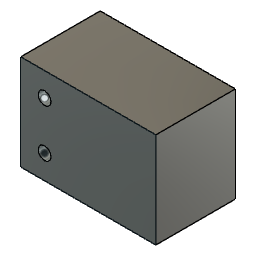
X-AxisLimitSwitchBlock v2 (Autodesk Fusion 360 design; units mm, degrees)
Autodesk Fusion 360 part; units mm, degrees
sketch "Sketch1" plane through (0, 0, 0) normal (0, 1, 0) x (1, 0, 0)
  line L0 (0, 0) -> (17, 0)
  line L1 (17, 0) -> (17, -10)
  line L2 (17, -10) -> (0, -10)
  line L3 (0, -10) -> (0, 0)
  dimension "d1" = 17
  dimension "d2" = 10
  constraint horizontal L0
  constraint vertical L1
  constraint horizontal L2
  constraint vertical L3
  constraint coincident L0.start L3.end
  measures "d1" distance of L0.start L0.end
  measures "d2" distance of L0.start L2.end
extrude "Extrude1" add sketch "Sketch1" along normal blind 12
sketch "Sketch2" plane through (0, 0, 10) normal (0, 0, 1) x (1, 0, 0)
  line L0 (0, 0) -> (17, 0)
  line L1 (17, 0) -> (17, 12)
  line L2 (17, 12) -> (0, 12)
  line L3 (0, 12) -> (0, 0)
  point P0 (3, 3)
  point P1 (3, 9)
  dimension "d5" = 3
  dimension "d6" = 3
  dimension "d7" = 6
  measures "d5" distance of L0 P0
  measures "d6" distance of L3 P0
  measures "d7" distance of P0 P1
hole "Hole1" at (3, 3, 10) direction (0, 0, -1) diameter 1.6 depth 5 tip angle 118
hole "Hole2" at (3, 9, 10) direction (0, 0, -1) diameter 1.6 depth 5 tip angle 118
